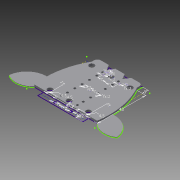
# Autodesk Inventor part: Piece
Saved by Autodesk Inventor 2014 SP1 (Build 180222100, 222)
## iProperties
Created: 2015-03-21
Part Number: Piece
Material: Generic
Document SubType Name: Modeling
Designer: Erin
Density: 1 g/cm^3
Appearance: Default
Author: Erin
Autodesk Inventor part; units mm, degrees
ref_plane "YZ Plane" through (0, 0, 0) normal (1, 0, 0) x (0, 1, 0)
ref_plane "XZ Plane" through (0, 0, 0) normal (0, 1, 0) x (-1, 0, 0)
ref_plane "XY Plane" through (0, 0, 0) normal (0, 0, 1) x (1, 0, 0)
sketch "Block1" plane through (0, 0, 0) normal (0, 0, 1) x (1, 0, 0)
  line L0 (22.5674, 54.9733) -> (22.5674, 26.9733) construction
  line L1 (62.5674, 54.9733) -> (62.5674, 26.9733) construction
  line L2 (42.5674, 54.9733) -> (42.5674, 26.9733) construction
  arc A0 (22.5674, 54.9733) -> (16.0189, 31.9733) centre (39.6923, 37.6653) ccw
  arc A1 (69.116, 31.9733) -> (62.5674, 54.9733) centre (45.4425, 37.6653) ccw
  line L3 (67.5674, 31.9733) -> (69.116, 31.9733)
  line L4 (22.5674, 54.9733) -> (62.5674, 54.9733)
  arc A2 (3.175, 28.049) -> (16.0189, 31.9733) centre (7.7246, 36.1392) ccw
  arc A3 (15.3685, 38.7512) -> (3.175, 28.049) centre (13.5542, 28.5209) ccw
  arc A4 (69.116, 31.9733) -> (81.9598, 28.049) centre (77.4102, 36.1392) ccw
  arc A5 (81.9598, 28.049) -> (69.7664, 38.7512) centre (71.5807, 28.5209) ccw
  line L5 (17.5674, 54.9733) -> (67.5674, 54.9733) construction
  line L6 (67.5674, 54.9733) -> (67.5674, 31.9733) construction
  line L7 (67.5674, 31.9733) -> (16.0189, 31.9733)
  line L8 (17.5674, 31.9733) -> (17.5674, 54.9733) construction
  line L9 (22.5674, 31.9733) -> (62.5674, 31.9733)
  line L10 (62.5674, 31.9733) -> (62.5674, 26.9733)
  line L11 (62.5674, 26.9733) -> (22.5674, 26.9733)
  line L12 (22.5674, 26.9733) -> (22.5674, 31.9733)
  circle A6 centre (35.5674, 51.6287) radius 1
  circle A7 centre (49.5674, 51.6287) radius 1
  line L13 (22.5674, 29.4733) -> (62.5674, 29.4733) construction
  circle A8 centre (35.5674, 29.4733) radius 1
  circle A9 centre (49.5674, 29.4733) radius 1
  point P0 (42.5377, 37.3132)
  point P1 (42.5674, 31.9733)
  point P2 (42.5674, 31.9733)
  point P3 (17.5674, 26.9733)
  point P4 (67.5674, 26.9733)
  dimension "d0" = 23
  dimension "d1" = 5
  dimension "d2" = 40
  dimension "d3" = 2
  dimension "d4" = 2
  dimension "d5" = 7
  dimension "d6" = 7
  dimension "d7" = 2
  dimension "d8" = 2
  dimension "d9" = 7
  dimension "d10" = 7
  measures "d0" distance of L5.end L3.start
  measures "d1" distance of L9.end L1.end
  measures "d2" distance of L9.start L9.end
  measures "d3" diameter of A6
  measures "d4" diameter of A7
  measures "d5" distance from line of A6.centre L2
  measures "d6" distance from line of A7.centre L2
  measures "d7" diameter of A8
  measures "d8" diameter of A9
  measures "d9" distance from line of A8.centre L2
  measures "d10" distance from line of A9.centre L2
sketch "Sketch1" plane through (0, 0, 0) normal (0, 0, 1) x (1, 0, 0)
  line L0 (-20, 21.5) -> (-20, -26.5) construction
  line L1 (20, 21.5) -> (20, -26.5) construction
  line L2 (0, 21.5) -> (0, -26.5) construction
  arc A0 (-20, 21.5) -> (-27.7782, -21.5) centre (37.6183, -11.126) ccw
  arc A1 (27.7782, -21.5) -> (20, 21.5) centre (-37.6183, -11.126) ccw
  line L3 (25, -21.5) -> (27.7782, -21.5)
  line L4 (-20, 21.5) -> (20, 21.5)
  line L5 (-25, 21.5) -> (25, 21.5) construction
  line L6 (25, 21.5) -> (25, -21.5) construction
  line L7 (25, -21.5) -> (-27.7782, -21.5)
  line L8 (-25, -21.5) -> (-25, 21.5) construction
  line L9 (-20, -21.5) -> (20, -21.5)
  line L10 (20, -21.5) -> (20, -26.5)
  line L11 (20, -26.5) -> (-20, -26.5)
  line L12 (-20, -26.5) -> (-20, -21.5)
  circle A2 centre (-7, 18.1554) radius 1
  circle A3 centre (7, 18.1554) radius 1
  line L13 (-20, -24) -> (20, -24) construction
  circle A4 centre (-7, -24) radius 1
  circle A5 centre (7, -24) radius 1
  circle A6 centre (-17, -18.5) radius 2.25
  circle A7 centre (17, -18.5) radius 2.25
  circle A8 centre (0, -18.5) radius 2.25
  line L14 (-25, 0) -> (25, 0) construction
  line L15 (-20, 21.5) -> (20, 21.5)
  line L16 (20, 21.5) -> (20, 26.5)
  line L17 (20, 26.5) -> (-20, 26.5)
  line L18 (-20, 26.5) -> (-20, 21.5)
  line L19 (-7, 18.1554) -> (-7, 26.5) construction
  line L20 (-7, 21.5) -> (-9.8868, 26.5)
  line L21 (-9.8868, 26.5) -> (-4.1132, 26.5)
  line L22 (-4.1132, 26.5) -> (-7, 21.5)
  circle A9 centre (-7, 0) radius 1
  circle A10 centre (7, 0) radius 1
  circle A11 centre (-7, -18.1554) radius 1
  circle A12 centre (7, -18.1554) radius 1
  arc A13 (-47.7296, -24) -> (-27.7782, -21.5) centre (-39.1631, -11.5041) ccw
  arc A14 (-28.5398, -8.4011) -> (-47.7296, -24) centre (-30.1563, -26.0155) ccw
  arc A15 (27.7782, -21.5) -> (47.7296, -24) centre (39.1631, -11.5041) ccw
  arc A16 (47.7296, -24) -> (28.5398, -8.4011) centre (30.1563, -26.0155) ccw
  point P0 (0, 0)
  point P1 (0, -21.5)
  point P2 (0, -21.5)
  point P3 (-27.9814, 24.963)
  point P4 (27.9814, 24.963)
  point P5 (0, -2.5)
  point P6 (0, 0)
  dimension "d12" = 43
  dimension "d13" = 5
  dimension "d14" = 40
  dimension "d15" = 2
  dimension "d16" = 2
  dimension "d17" = 7
  dimension "d18" = 7
  dimension "d19" = 2
  dimension "d20" = 2
  dimension "d21" = 7
  dimension "d22" = 7
  dimension "d24" = 4.5
  dimension "d25" = 4.5
  dimension "d26" = 3
  dimension "d27" = 3
  dimension "d28" = 3
  dimension "d29" = 3
  dimension "d34" = 4.5
  dimension "d35" = 3
  dimension "d38" = 5
  dimension "d39" = 30
  dimension "d40" = 30
  dimension "d45" = 3.3446
  dimension "d46" = 3.3446
  dimension "d47" = 2
  dimension "d48" = 2
  dimension "d49" = 7
  dimension "d50" = 7
  constraints: 46 end point, 17 centre point, 14 point on line, 13 point on circle, 9 midpoint, 8 parallel, 7 symmetric about line, 5 perpendicular, 4 horizontal, 2 collinear, 1 coincident, 1 vertical, 5 other
  measures "d12" distance of L5.end L3.start
  measures "d13" distance of L9.end L1.end
  measures "d14" distance of L9.start L9.end
  measures "d15" diameter of A2
  measures "d16" diameter of A3
  measures "d17" distance from line of L19.start L2
  measures "d18" distance from line of A3.centre L2
  measures "d19" diameter of A4
  measures "d20" diameter of A5
  measures "d21" distance from line of A4.centre L2
  measures "d22" distance from line of A5.centre L2
  measures "d24" diameter of A6
  measures "d25" diameter of A7
  measures "d26" distance from line of A6.centre L0
  measures "d27" distance from line of A7.centre L1
  measures "d28" distance from line of A6.centre L9
  measures "d29" distance from line of A7.centre L7
  measures "d34" diameter of A8
  measures "d35" distance from line of A8.centre L9
  measures "d38" distance of L16.end L15.end
  measures "d39" angle of L19 L20
  measures "d40" angle of L19 L22
  measures "d45" distance from line of L19.start L5
  measures "d46" distance from line of A3.centre L5
  measures "d47" diameter of A9
  measures "d48" diameter of A10
  measures "d49" distance from line of L2 A9.centre
  measures "d50" distance from line of A10.centre L2
extrude "Extrusion1" add sketch "Sketch1" along normal blind 2 contours L4 A1 L3 L7 A0 | A6 | A7 | A8 | A9 | A10
extrude "Extrusion2" add sketch "Sketch1" along normal blind 0.6 contours L4 A1 L3 L7 A0 | A2 | A3 | A6 | A7 | A8 | A9 | A10 | A11 | A12
mirror "Mirror1" about plane through (0, 0, 0) normal (1, 0, 0) of "Extrusion2"
extrude "Extrusion3" cut sketch "Sketch1" along normal blind 5 contours A6 | A7 | A8
mirror "Mirror2" about plane through (0, 0, 0) normal (0, 1, 0) of "Extrusion3"
extrude "Extrusion4" add sketch "Sketch1" along normal blind 2 contours L18 L17 L20 L4 | L22 L17 L16 L4 | L20 L17 L22
extrude "Extrusion5" cut sketch "Sketch1" along normal blind 5 contours L20 L17 L22
extrude "Extrusion7" add sketch "Sketch1" along normal blind 0.6 contours A0 A13 A14
mirror "Mirror3" about plane through (0, 0, 0) normal (1, 0, 0) of "Extrusion5", "Extrusion7"
fillet "Fillet1" radius 3 2 edges at (-20, 26.5, 1) (20, 26.5, 1)
extrude "Extrusion8" cut sketch "Sketch1" along normal blind 10 contours A9 | A10
pattern_linear "Rectangular Pattern1" count 3 spacing 6.5 along (0, 1, 0) count 3 spacing 6.5 along (0, -1, 0) of "Extrusion8"
equation "\"d3\" = d11"
equation "\"d4\" = d11"
equation "\"d7\" = d11"
equation "\"d8\" = d11"
equation "\"d15\" = fishing"
equation "\"d16\" = fishing"
equation "\"d19\" = fishing"
equation "\"d20\" = fishing"
equation "\"d47\" = fishing"
equation "\"d48\" = fishing"
equation "\"d56\" = 2 * layer"
equation "\"d11\" = 2"
equation "\"d23\" = 2"
equation "\"fishing\" = 2"
equation "\"layer\" = 0.3"
body "Solid1"
